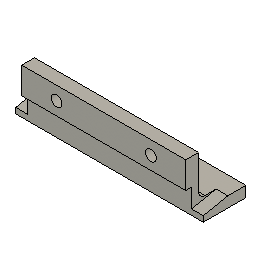
Bracket (Autodesk Fusion 360 design; units mm, degrees)
Autodesk Fusion 360 part; units mm, degrees
sketch "Sketch1" plane through (0, 0, 0) normal (0, 1, 0) x (1, 0, 0)
  line L0 (44, -10) -> (-44, -10)
  line L1 (-44, -10) -> (-44, 10)
  line L2 (-44, 10) -> (44, 10)
  line L3 (44, 10) -> (44, -10)
  line L4 (44, -10) -> (-44, 10) construction
  line L5 (-44, -10) -> (44, 10) construction
  dimension "d1" = 88
  dimension "d2" = 20
  constraint horizontal L0
  constraint perpendicular L0 L1
  constraint parallel L0 L2
  constraint parallel L1 L3
  constraint coincident L4 origin
  constraint coincident L5 origin
  measures "d1" distance of L1.end L2.end
  measures "d2" distance of L0.end L1.end
extrude "Extrude1" add sketch "Sketch1" along normal blind 5
sketch "Sketch2" plane through (0, 5, 0) normal (0, 1, 0) x (-1, 0, 0)
  line L0 (-44, -10) -> (44, -10)
  line L1 (44, -10) -> (44, 10)
  line L2 (44, 10) -> (-44, 10)
  line L3 (-44, 10) -> (-44, -10)
  line L4 (44, 10) -> (44, 6.75)
  line L5 (44, 6.75) -> (-44, 6.75)
  dimension "d5" = 3.25
  constraint coincident L1.end L2.start
  constraint perpendicular L2 L4
  constraint coincident L3 L5.end
  constraint perpendicular L3 L5
  measures "d5" distance of L1.end L4.end
extrude "Extrude2" add sketch "Sketch2" along normal blind 19 contours L1 L2 L3 L4 L5
sketch "Sketch3" plane through (0, 0, 10) normal (0, 0, 1) x (1, 0, 0)
  line L0 (-44, 0) -> (44, 0)
  line L1 (44, 0) -> (44, 24)
  line L2 (44, 24) -> (-44, 24)
  line L3 (-44, 24) -> (-44, 0)
  line L4 (-44, 24) -> (44, 24)
  line L5 (44, 24) -> (44, 11.5)
  line L6 (44, 11.5) -> (-44, 11.5)
  line L7 (-44, 11.5) -> (-44, 24)
  dimension "d8" = 12.5
  constraint horizontal L4
  constraint vertical L5
  constraint horizontal L6
  constraint vertical L7
  constraint coincident L2.end L3.start
  measures "d8" distance of L2.end L6.end
extrude "Extrude3" add sketch "Sketch3" along normal blind 2.75 contours L1 L2 L3 L4 L5 L6 L7
sketch "Sketch4" plane through (44, 0, 0) normal (1, 0, 0) x (0, 0, -1)
  line L0 (-10, 0) -> (10, 0)
  line L1 (10, 0) -> (10, 5)
  line L2 (10, 5) -> (-6.75, 5)
  line L3 (-6.75, 5) -> (-6.75, 24)
  line L4 (-6.75, 24) -> (-12.75, 24)
  line L5 (-12.75, 24) -> (-12.75, 11.5)
  line L6 (-12.75, 11.5) -> (-10, 11.5)
  line L7 (-10, 11.5) -> (-10, 0)
  line L8 (-6.75, 5) -> (-10, 5)
  constraint coincident L2.end L3.start
  constraint coincident L7 L8.end
  constraint perpendicular L7 L8
extrude "Extrude4" cut sketch "Sketch4" against normal blind 5.5 contours L3 L4 L5 L6 L7 L8
sketch "Sketch5" plane through (-44, 0, 0) normal (-1, 0, 0) x (0, 0, 1)
  line L0 (-10, 0) -> (10, 0)
  line L1 (10, 0) -> (10, 11.5)
  line L2 (10, 11.5) -> (12.75, 11.5)
  line L3 (12.75, 11.5) -> (12.75, 24)
  line L4 (12.75, 24) -> (6.75, 24)
  line L5 (6.75, 24) -> (6.75, 5)
  line L6 (6.75, 5) -> (-10, 5)
  line L7 (-10, 5) -> (-10, 0)
  line L8 (6.75, 5) -> (10, 5)
  point P0 (10, 5)
  constraint coincident L5.end L6.start
  constraint coincident P0 L8.end
extrude "Extrude5" cut sketch "Sketch5" against normal blind 5.5 contours L1 L2 L3 L4 L5 L8
sketch "Sketch6" plane through (-44, 0, 0) normal (-1, 0, 0) x (0, 0, 1)
  line L0 (10, 5) -> (-10, 5)
  line L1 (-10, 5) -> (-10, 0)
  line L2 (-10, 0) -> (10, 0)
  line L3 (10, 0) -> (10, 5)
  line L4 (10, 0) -> (10, 2.65)
  line L5 (10, 5) -> (0, 5)
  line L6 (0, 5) -> (10, 2.65)
  dimension "d15" = 2.65
  dimension "d16" = 10
  constraint coincident L2.end L3.start
  constraint perpendicular L2 L4
  constraint coincident L0.start L3.end
  constraint perpendicular L3 L5
  measures "d15" distance of L2.end L4.end
  measures "d16" distance of L0.start L5.end
extrude "Extrude6" cut sketch "Sketch6" against normal blind 5.5 contours L0 L3 L5 L6
sketch "Sketch7" plane through (44, 0, 0) normal (1, 0, 0) x (0, 0, -1)
  line L0 (10, 5) -> (-10, 5)
  line L1 (-10, 5) -> (-10, 0)
  line L2 (-10, 0) -> (10, 0)
  line L3 (10, 0) -> (10, 5)
  line L4 (-10, 0) -> (-10, 2.65)
  line L5 (-10, 5) -> (0, 5)
  line L6 (-10, 5) -> (1.5, 5)
  line L7 (1.5, 5) -> (-10, 2.65)
  point P0 (0, 5)
  point P1 (0, 5)
  dimension "d19" = 2.65
  dimension "d48" = 11.5
  constraint coincident L1.end L2.start
  constraint perpendicular L2 L4
  constraint coincident L0.end L1.start
  constraint coincident P1 P0
  constraint perpendicular L1 L6
  measures "d19" distance of L1.end L4.end
  measures "d48" distance of L0.end L6.end
extrude "Extrude7" cut sketch "Sketch7" against normal blind 5.5
fillet "Fillet1" radius 3 1 edges at (0, 5, 6.75)
sketch "Sketch9" plane through (0, 0, 12.75) normal (0, 0, -1) x (-1, 0, 0)
  line L0 (-38.5, 8) -> (38.5, 8)
  line L1 (38.5, 8) -> (38.5, 24)
  line L2 (38.5, 24) -> (-38.5, 24)
  line L3 (-38.5, 24) -> (-38.5, 8)
  circle A0 centre (22.15, 17.65) radius 2.5
  circle A1 centre (-22.15, 17.65) radius 2.5
  line L4 (38.5, 24) -> (-38.5, 24)
  line L5 (38.5, 8) -> (38.5, 24)
  line L6 (38.5, 24) -> (38.5, 11.5)
  line L7 (-38.5, 11.5) -> (-38.5, 24)
  line L8 (-38.5, 24) -> (38.5, 24)
  line L9 (38.5, 11.5) -> (-38.5, 11.5)
  dimension "d27" = 5
  dimension "d28" = 6.35
  dimension "d29" = 5
  dimension "d30" = 6.35
  dimension "d31" = 44.3
  dimension "d32" = 16.35
  measures "d27" diameter of A0
  measures "d28" distance of L2 A0.centre
  measures "d29" diameter of A1
  measures "d30" distance of A1.centre L4
  measures "d31" distance of A0.centre A1.centre
  measures "d32" distance of A0.centre L5
sketch "Sketch10" plane through (0, 0, 12.75) normal (0, 0, -1) x (-1, 0, 0)
sketch "Sketch11" plane through (0, 0, 6.75) normal (0, 0, -1) x (-1, 0, 0)
  line L0 (-38.5, 8) -> (38.5, 8)
  line L1 (38.5, 8) -> (38.5, 24)
  line L2 (38.5, 24) -> (-38.5, 24)
  line L3 (-38.5, 24) -> (-38.5, 8)
  circle A0 centre (-22.15, 17.65) radius 2.875
  circle A1 centre (22.15, 17.65) radius 2.875
  point P0 (-22.15, 17.65)
  point P1 (22.15, 17.65)
  dimension "d33" = 5.75
  dimension "d34" = 5.75
  constraint coincident P0 A0.centre
  constraint coincident P1 A1.centre
  measures "d33" diameter of A0
  measures "d34" diameter of A1
loft "Loft1" cut profiles "Sketch11", "Sketch9" section 1 contours A0 section 2 contours A1
loft "Loft2" cut profiles "Sketch9", "Sketch11" section 1 contours A0 section 2 contours A1
sketch "Sketch12" plane through (0, 5, 0) normal (0, 1, 0) x (-1, 0, 0)
  line L0 (38.5, 3.75) -> (-38.5, 3.75)
  line L1 (-38.5, 3.75) -> (-38.5, -10)
  line L2 (-38.5, -10) -> (44, -10)
  line L3 (44, -10) -> (44, 0)
  line L4 (44, 0) -> (38.5, 0)
  line L5 (38.5, 0) -> (38.5, 3.75)
sketch "Sketch13" plane through (0, 0, 12.75) normal (0, 0, -1) x (1, 0, 0)
sketch "Sketch14" plane through (0, 5, 0) normal (0, 1, 0) x (-1, 0, 0)
  line L0 (38.5, 3.75) -> (-38.5, 3.75)
  line L1 (-38.5, 3.75) -> (-38.5, -10)
  line L2 (-38.5, -10) -> (44, -10)
  line L3 (44, -10) -> (44, 0)
  line L4 (44, 0) -> (38.5, 0)
  line L5 (38.5, 0) -> (38.5, 3.75)
  line L6 (22.15, -1.575) -> (-22.15, -1.575)
  line L7 (25.65, 0.05) -> (25.65, -3.2)
  line L8 (18.65, -3.2) -> (18.65, 0.05)
  line L9 (18.65, 3.55) -> (25.65, -6.7) construction
  line L10 (25.65, 3.55) -> (18.65, -6.7) construction
  arc A0 (18.65, -3.2) -> (22.15, -6.7) centre (22.15, -3.2) ccw
  arc A1 (22.15, -6.7) -> (25.65, -3.2) centre (22.15, -3.2) ccw
  arc A2 (25.65, 0.05) -> (22.15, 3.55) centre (22.15, 0.05) ccw
  arc A3 (22.15, 3.55) -> (18.65, 0.05) centre (22.15, 0.05) ccw
  line L11 (-18.65, 0.05) -> (-18.65, -3.2)
  line L12 (-25.65, -3.2) -> (-25.65, 0.05)
  line L13 (-25.65, 3.55) -> (-18.65, -6.7) construction
  line L14 (-18.65, 3.55) -> (-25.65, -6.7) construction
  arc A4 (-22.15, -6.7) -> (-18.65, -3.2) centre (-22.15, -3.2) ccw
  arc A5 (-25.65, -3.2) -> (-22.15, -6.7) centre (-22.15, -3.2) ccw
  arc A6 (-22.15, 3.55) -> (-25.65, 0.05) centre (-22.15, 0.05) ccw
  arc A7 (-18.65, 0.05) -> (-22.15, 3.55) centre (-22.15, 0.05) ccw
  point P0 (22.15, -1.575)
  point P1 (-22.15, -1.575)
  dimension "d35" = 44.3
  dimension "d36" = 21.85
  dimension "d37" = 7
  dimension "d38" = 10.25
  dimension "d40" = 3.5
  dimension "d41" = 7
  dimension "d42" = 10.25
  dimension "d43" = 3.5
  constraint horizontal L6
  constraint parallel L7 L8
  constraint coincident L9 P0
  constraint coincident L10 P0
  constraint coincident P0 L6.start
  constraint coincident L10.end L8
  constraint tangent L8 A0
  constraint coincident L9.end L7
  constraint tangent L7 A1
  constraint equal A0 A1
  constraint coincident A0.end A1.start
  constraint coincident L10.start L7
  constraint tangent L7 A2
  constraint equal A0 A2
  constraint coincident L9.start L8
  constraint tangent L8 A3
  constraint equal A0 A3
  constraint coincident A2.end A3.start
  constraint parallel L11 L12
  constraint coincident L13 P1
  constraint coincident L14 P1
  constraint coincident P1 L6.end
  constraint coincident L13.end L11
  constraint tangent L11 A4
  constraint coincident L14.end L12
  constraint tangent L12 A5
  constraint equal A4 A5
  constraint coincident A4.start A5.end
  constraint coincident L13.start L12
  constraint tangent L12 A6
  constraint equal A4 A6
  constraint coincident L14.start L11
  constraint tangent L11 A7
  constraint equal A4 A7
  constraint coincident A6.start A7.end
  measures "d35" distance of P0 P1
  measures "d36" distance of L3 P0
  measures "d37" distance of L9.end L10.end
  measures "d38" distance of L10.start L9.end
  measures "d40" radius of A0
  measures "d41" distance of L13.end L14.end
  measures "d42" distance of L14.start L13.end
  measures "d43" radius of A4
extrude "Extrude8" cut sketch "Sketch14" against normal blind 5 contours L7 L8 A0 A1 A2 A3 | L11 L12 A4 A5 A6 A7
extrude "Extrude9" add sketch "Sketch7" against normal blind 5.5 contours L0 L1 L2 L3 L4 L7
